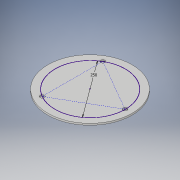
# Autodesk Inventor part: Fußßß
Saved by Autodesk Inventor 2019 (Build 230136000, 136)
## iProperties
Created: 2018-08-07
Part Number: Fußßß
Material: Generic
Document SubType Name: Modeling
Designer: Julia
Density: 1 g/cm^3
Appearance: Default
Author: Julia
Autodesk Inventor part; units mm, degrees
ref_plane "YZ Plane" through (0, 0, 0) normal (1, 0, 0) x (0, 1, 0)
ref_plane "XZ Plane" through (0, 0, 0) normal (0, 1, 0) x (-1, 0, 0)
ref_plane "XY Plane" through (0, 0, 0) normal (0, 0, 1) x (1, 0, 0)
sketch "Sketch6" plane through (0, 0, 0) normal (0, 1, 0) x (-1, 0, 0)
  circle A0 centre (0, 0) radius 150
  dimension "d17" = 300
  constraints: 1 centre point, 1 coincident
  measures "d17" diameter of A0
extrude "Extrusion3" add sketch "Sketch6" along normal blind 6
sketch "Sketch7" plane through (0, 6, 0) normal (0, 1, 0) x (1, 0, 0)
  circle A0 centre (0, 0) radius 125
  line L0 (125, 0) -> (-62.5, 108.2532) construction
  line L1 (-62.5, 108.2532) -> (-62.5, -108.2532) construction
  line L2 (-62.5, -108.2532) -> (125, 0) construction
  dimension "d20" = 250
  constraints: 6 end point, 3 point on circle, 2 equal length, 1 centre point, 1 coincident, 1 horizontal alignment
  measures "d20" diameter of A0
hole "Hole2" at (125, 6, 0) direction (0, -1, 0) diameter 15 depth 4
hole "Hole3" at (-62.5, 6, 108.2532) direction (0, -1, 0) diameter 15 depth 4
hole "Hole4" at (-62.5, 6, -108.2532) direction (0, -1, 0) diameter 15 depth 4
body "Solid2"
